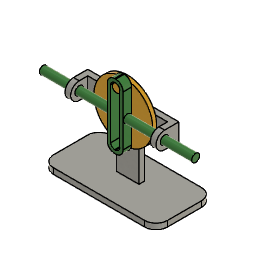
Scotch yoke v1 (Autodesk Fusion 360 design; units mm, degrees)
Autodesk Fusion 360 part; units mm, degrees
sketch "Sketch1" plane through (0, 0, 0) normal (0, 0, 1) x (1, 0, 0)
  line L0 (-40, 25) -> (40, 25)
  line L1 (50, 15) -> (50, -15)
  line L2 (40, -25) -> (-40, -25)
  line L3 (-50, -15) -> (-50, 15)
  arc A0 (-40, 25) -> (-50, 15) centre (-40, 15) ccw
  arc A1 (50, 15) -> (40, 25) centre (40, 15) ccw
  arc A2 (40, -25) -> (50, -15) centre (40, -15) ccw
  arc A3 (-50, -15) -> (-40, -25) centre (-40, -15) ccw
  dimension "d1" = 10
  constraint horizontal L0
  constraint vertical L1
  constraint horizontal L2
  constraint vertical L3
  constraint tangent L0 A0
  constraint tangent L3 A0
  constraint tangent L0 A1
  constraint tangent L1 A1
  constraint equal A0 A1
  constraint tangent L1 A2
  constraint tangent L2 A2
  constraint equal A0 A2
  constraint tangent L2 A3
  constraint tangent L3 A3
  constraint equal A0 A3
  measures "d1" radius of A0
extrude "Extrude1" add sketch "Sketch1" along normal blind 5 makes body 1
sketch "Sketch2" plane through (0, 0, 5) normal (0, 0, 1) x (-1, 0, 0)
  arc A0 (40, -25) -> (50, -15) centre (40, -15) ccw
  line L0 (50, -15) -> (50, 15)
  arc A1 (50, 15) -> (40, 25) centre (40, 15) ccw
  line L1 (40, 25) -> (-40, 25)
  arc A2 (-40, 25) -> (-50, 15) centre (-40, 15) ccw
  line L2 (-50, 15) -> (-50, -15)
  arc A3 (-50, -15) -> (-40, -25) centre (-40, -15) ccw
  line L3 (-40, -25) -> (40, -25)
  line L4 (10, -5) -> (-10, -5)
  line L5 (-10, -5) -> (-10, 0)
  line L6 (-10, 0) -> (10, 0)
  line L7 (10, 0) -> (10, -5)
  constraint horizontal L4
  constraint vertical L5
  constraint horizontal L6
  constraint vertical L7
extrude "Extrude2" add sketch "Sketch2" along normal blind 60 contours L4 L5 L6 L7 bodies 1
sketch "Sketch3" plane through (10, 0, 0) normal (1, 0, 0) x (0, 1, 0)
  line L0 (0, 5) -> (5, 5)
  line L1 (5, 5) -> (5, 65)
  line L2 (5, 65) -> (0, 65)
  line L3 (0, 65) -> (0, 5)
  line L4 (0, 65) -> (5, 65)
  line L5 (5, 65) -> (5, 50)
  line L6 (5, 50) -> (0, 50)
  line L7 (0, 50) -> (0, 65)
  constraint horizontal L4
  constraint vertical L5
  constraint horizontal L6
  constraint vertical L7
  constraint coincident L1 L5.end
  constraint coincident L2.end L3.start
extrude "Extrude3" add sketch "Sketch3" along normal blind 30 contours L1 L2 L3 L4 L5 L6 L7 bodies 1
sketch "Sketch4" plane through (-10, 0, 0) normal (-1, 0, 0) x (0, -1, 0)
  line L0 (-5, 5) -> (0, 5)
  line L1 (0, 5) -> (0, 65)
  line L2 (0, 65) -> (-5, 65)
  line L3 (-5, 65) -> (-5, 5)
  line L4 (-5, 65) -> (0, 65)
  line L5 (0, 65) -> (0, 50)
  line L6 (0, 50) -> (-5, 50)
  line L7 (-5, 50) -> (-5, 65)
  constraint horizontal L4
  constraint vertical L5
  constraint horizontal L6
  constraint vertical L7
  constraint coincident L1 L5.end
  constraint coincident L2.end L3.start
extrude "Extrude4" add sketch "Sketch4" along normal blind 30 contours L1 L2 L3 L4 L5 L6 L7 bodies 1
sketch "Sketch5" plane through (0, 0, 0) normal (0, -1, 0) x (1, 0, 0)
  line L0 (-10, 5) -> (10, 5)
  line L1 (10, 5) -> (10, 50)
  line L2 (10, 50) -> (40, 50)
  line L3 (40, 50) -> (40, 65)
  line L4 (40, 65) -> (-40, 65)
  line L5 (-40, 65) -> (-40, 50)
  line L6 (-40, 50) -> (-10, 50)
  line L7 (-10, 50) -> (-10, 5)
  line L8 (-40, 65) -> (-35, 65)
  line L9 (-35, 65) -> (-35, 50)
  line L10 (-35, 50) -> (-40, 50)
  line L11 (-40, 50) -> (-40, 65)
  line L12 (35, 65) -> (40, 65)
  line L13 (40, 65) -> (40, 50)
  line L14 (40, 50) -> (35, 50)
  line L15 (35, 50) -> (35, 65)
  constraint horizontal L8
  constraint vertical L9
  constraint horizontal L10
  constraint vertical L11
  constraint coincident L6 L9.end
  constraint coincident L4.end L5.start
  constraint horizontal L12
  constraint vertical L13
  constraint horizontal L14
  constraint vertical L15
  constraint coincident L2.end L3.start
  constraint coincident L4 L12.start
extrude "Extrude5" add sketch "Sketch5" along normal blind 15 contours L4 L5 L6 L8 L9 L10 L11 | L2 L3 L4 L12 L13 L14 L15 bodies 1
fillet "Fillet1" radius 7.5 4 edges at (-37.5, -15, 65) (-37.5, -15, 50) (37.5, -15, 65) (37.5, -15, 50) on bodies 1
sketch "Sketch6" plane through (40, 0, 0) normal (1, 0, 0) x (0, 1, 0)
  arc A0 (-7.5, 65) -> (-7.5, 50) centre (-7.5, 57.5) ccw
  line L0 (-7.5, 50) -> (5, 50)
  line L1 (5, 50) -> (5, 65)
  line L2 (5, 65) -> (-7.5, 65)
  circle A1 centre (-7.5, 57.5) radius 3.8079
  constraint concentric A0 A1
extrude "Extrude6" cut sketch "Sketch6" against normal blind 90 contours A1 bodies 1
sketch "Sketch7" plane through (0, 0, 0) normal (0, -1, 0) x (1, 0, 0)
  line L0 (35, 50) -> (35, 65)
  line L1 (35, 65) -> (-35, 65)
  line L2 (-35, 65) -> (-35, 50)
  line L3 (-35, 50) -> (-10, 50)
  line L4 (-10, 50) -> (-10, 5)
  line L5 (-10, 5) -> (10, 5)
  line L6 (10, 5) -> (10, 50)
  line L7 (10, 50) -> (35, 50)
  line L8 (0, 65) -> (0, 57.5)
  circle A0 centre (0, 57.5) radius 3.2016
  dimension "d16" = 7.5
  constraint midpoint L1 L8.start
  constraint perpendicular L1 L8
  constraint coincident L8.end A0.centre
  measures "d16" distance of L8.start L8.end
extrude "Extrude7" cut sketch "Sketch7" against normal blind 15 contours A0 bodies 1
sketch "Sketch8" plane through (0, 0, 0) normal (0, -1, 0) x (1, 0, 0)
  circle A0 centre (0, 57.5) radius 3.2016
  line L0 (35, 50) -> (35, 65)
  line L1 (35, 65) -> (-35, 65)
  line L2 (-35, 65) -> (-35, 50)
  line L3 (-35, 50) -> (-10, 50)
  line L4 (-10, 50) -> (-10, 5)
  line L5 (-10, 5) -> (10, 5)
  line L6 (10, 5) -> (10, 50)
  line L7 (10, 50) -> (35, 50)
sketch "Sketch9" plane through (0, 0, 0) normal (0, 1, 0) x (1, 0, 0)
  circle A0 centre (0, -57.5) radius 25.8312
extrude "Extrude1'" add sketch "Sketch9" against normal blind 3.5 separate body makes body 2 in component "Rotational"
move_body "Move1" bodies 2 to x (1, 0, 0) y (0, 1, 0) z (0, 0, 1) at (0, -0.25, 0) in component "Rotational"
sketch "Sketch10" plane through (0, -0.25, 0) normal (0, 1, 0) x (-1, 0, 0)
  circle A0 centre (0, 57.5) radius 25.8312
  circle A1 centre (0, 57.5) radius 3.0806
  constraint concentric A0 A1
extrude "Extrude8" add sketch "Sketch8" against normal blind 5.1 contours A0 bodies 1
sketch "Sketch11" plane through (0, 5.1, 0) normal (0, 1, 0) x (-1, 0, 0)
  circle A0 centre (0, 57.5) radius 3.2016
  circle A1 centre (0, 57.5) radius 4.9119
  constraint concentric A0 A1
extrude "Extrude9" add sketch "Sketch11" along normal blind 0.5 contours A0 | A1 bodies 1
copy_body "Body->Comp1" bodies 1 removing the originals makes body 3 in component "Stand"
sketch "Sketch12" plane through (0, -3.75, 0) normal (0, -1, 0) x (1, 0, 0)
  circle A0 centre (0, 57.5) radius 25.8312
  circle A1 centre (0, 78) radius 3.6056
extrude "Extrude2'" add sketch "Sketch12" along normal blind 6 contours A1 bodies 2 in component "Rotational"
sketch "Sketch13" plane through (0, -3.75, 0) normal (0, -1, 0) x (1, 0, 0)
  circle A0 centre (0, 78) radius 3.6056
  circle A1 centre (0, 57.5) radius 25.8312
  line L0 (-0.4642, 83.0252) -> (0.4343, 83.0252)
  line L1 (3.9343, 79.5252) -> (3.9343, 35.4702)
  line L2 (0.4343, 31.9702) -> (-0.4642, 31.9702)
  line L3 (-3.9642, 35.4702) -> (-3.9642, 79.5252)
  arc A2 (-0.4642, 83.0252) -> (-3.9642, 79.5252) centre (-0.4642, 79.5252) ccw
  arc A3 (3.9343, 79.5252) -> (0.4343, 83.0252) centre (0.4343, 79.5252) ccw
  arc A4 (0.4343, 31.9702) -> (3.9343, 35.4702) centre (0.4343, 35.4702) ccw
  arc A5 (-3.9642, 35.4702) -> (-0.4642, 31.9702) centre (-0.4642, 35.4702) ccw
  line L4 (-0.4642, 86.0252) -> (0.4343, 86.0252)
  arc A6 (6.9343, 79.5252) -> (0.4343, 86.0252) centre (0.4343, 79.5252) ccw
  line L5 (6.9343, 79.5252) -> (6.9343, 35.4702)
  arc A7 (0.4343, 28.9702) -> (6.9343, 35.4702) centre (0.4343, 35.4702) ccw
  line L6 (0.4343, 28.9702) -> (-0.4642, 28.9702)
  arc A8 (-6.9642, 35.4702) -> (-0.4642, 28.9702) centre (-0.4642, 35.4702) ccw
  line L7 (-6.9642, 35.4702) -> (-6.9642, 79.5252)
  arc A9 (-0.4642, 86.0252) -> (-6.9642, 79.5252) centre (-0.4642, 79.5252) ccw
  dimension "d27" = 3.5
  dimension "d28" = 3
  constraint horizontal L0
  constraint vertical L1
  constraint horizontal L2
  constraint vertical L3
  constraint tangent L0 A2
  constraint tangent L3 A2
  constraint tangent L0 A3
  constraint tangent L1 A3
  constraint equal A2 A3
  constraint tangent L1 A4
  constraint tangent L2 A4
  constraint equal A2 A4
  constraint tangent L2 A5
  constraint tangent L3 A5
  constraint equal A2 A5
  measures "d27" radius of A2
extrude "Extrude1''" add sketch "Sketch13" along normal blind 7.5 separate body contours A1 A6 L5 A7 A8 L7 A9 | A1 L4 A6 A9 | A1 A7 L6 A8 makes body 4 in component "Linear"
sketch "Sketch14" plane through (6.9343, 0, 0) normal (1, 0, 0) x (0, 1, 0)
  line L0 (-3.75, 35.4702) -> (-3.75, 79.5252)
  line L1 (-3.75, 79.5252) -> (-11.25, 79.5252)
  line L2 (-11.25, 79.5252) -> (-11.25, 35.4702)
  line L3 (-11.25, 35.4702) -> (-3.75, 35.4702)
  circle A0 centre (-7.5026, 57.4977) radius 3.4911
extrude "Extrude2''" add sketch "Sketch14" along normal blind 60 contours A0 bodies 4 in component "Linear"
sketch "Sketch15" plane through (-6.9642, 0, 0) normal (-1, 0, 0) x (0, -1, 0)
  line L0 (3.75, 79.5252) -> (3.75, 35.4702)
  line L1 (3.75, 35.4702) -> (11.25, 35.4702)
  line L2 (11.25, 35.4702) -> (11.25, 79.5252)
  line L3 (11.25, 79.5252) -> (3.75, 79.5252)
  circle A0 centre (7.5, 57.5) radius 3.491
  dimension "d33" = 6.982
  measures "d33" diameter of A0
extrude "Extrude3'" add sketch "Sketch15" along normal blind 60 contours A0 bodies 4 in component "Linear"
component "Rotational" placed x (1, 0, 0) y (0, 1, 0) z (0, 0, 1) at (0, 0, 0)
component "Stand" placed x (1, 0, 0) y (0, 1, 0) z (0, 0, 1) at (0, 0, 0)
component "Linear" placed x (1, 0, 0) y (0, 1, 0) z (0, 0, 1) at (0, -0.02, 0)
